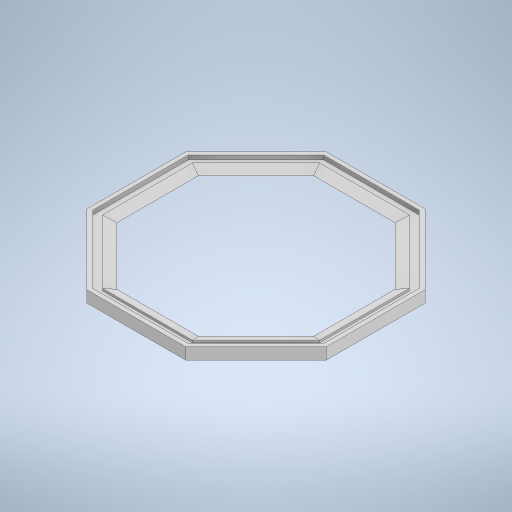
# Autodesk Inventor part: OV-PAM_ring_2
Saved by Autodesk Inventor 2024 (Build 280153000, 153)
## iProperties
Created: 2023-06-19
Part Number: OV-PAM_ring_2
Material: 일반
Document SubType Name: Modeling
Designer: jsw
Density: 1 g/cm^3
Appearance: 기본값
Author: jsw
Autodesk Inventor part; units mm, degrees
ref_plane "YZ Plane" through (0, 0, 0) normal (1, 0, 0) x (0, 1, 0)
ref_plane "XZ Plane" through (0, 0, 0) normal (0, 1, 0) x (-1, 0, 0)
sketch "스케치1" plane through (0, 0, 0) normal (0, 1, 0) x (-1, 0, 0)
  line L0 (-32.5919, 13.5) -> (-13.5, 32.5919)
  line L1 (-13.5, 32.5919) -> (13.5, 32.5919)
  line L2 (13.5, 32.5919) -> (32.5919, 13.5)
  line L3 (32.5919, 13.5) -> (32.5919, -13.5)
  line L4 (32.5919, -13.5) -> (13.5, -32.5919)
  line L5 (13.5, -32.5919) -> (-13.5, -32.5919)
  line L6 (-13.5, -32.5919) -> (-32.5919, -13.5)
  line L7 (-32.5919, -13.5) -> (-32.5919, 13.5)
  line L8 (34.9919, 14.4941) -> (34.9919, -14.4941)
  line L9 (34.9919, -14.4941) -> (14.4941, -34.9919)
  line L10 (14.4941, -34.9919) -> (-14.4941, -34.9919)
  line L11 (-14.4941, -34.9919) -> (-34.9919, -14.4941)
  line L12 (-34.9919, -14.4941) -> (-34.9919, 14.4941)
  line L13 (-34.9919, 14.4941) -> (-14.4941, 34.9919)
  line L14 (-14.4941, 34.9919) -> (14.4941, 34.9919)
  line L15 (14.4941, 34.9919) -> (34.9919, 14.4941)
  point P0 (0, 0)
  point P1 (0, 0)
  point P2 (0, 0)
  dimension "d0" = 27
  dimension "d1" = 2.4
  constraints: 32 end point, 2 coincident, 2 horizontal, 34 other
  measures "d0" distance of L2.end L3.end
  measures "d1" distance between parallel lines of L8 L3
extrude "돌출1" add sketch "스케치1" along normal blind 3.4 contours L0 L1 L2 L3 L4 L5 L6 L7 | L8 L9 L10 L11 L12 L13 L14 L15
sketch "스케치3" plane through (0, 0, 0) normal (0, -1, 0) x (1, 0, 0)
  line L0 (-13.5, 32.5919) -> (13.5, 32.5919)
  line L1 (13.5, 32.5919) -> (32.5919, 13.5)
  line L2 (32.5919, 13.5) -> (32.5919, -13.5)
  line L3 (32.5919, -13.5) -> (13.5, -32.5919)
  line L4 (13.5, -32.5919) -> (-13.5, -32.5919)
  line L5 (-13.5, -32.5919) -> (-32.5919, -13.5)
  line L6 (-32.5919, -13.5) -> (-32.5919, 13.5)
  line L7 (-32.5919, 13.5) -> (-13.5, 32.5919)
  line L8 (-13.9971, 33.7919) -> (13.9971, 33.7919)
  line L9 (13.9971, 33.7919) -> (33.7919, 13.9971)
  line L10 (33.7919, 13.9971) -> (33.7919, -13.9971)
  line L11 (33.7919, -13.9971) -> (13.9971, -33.7919)
  line L12 (13.9971, -33.7919) -> (-13.9971, -33.7919)
  line L13 (-13.9971, -33.7919) -> (-33.7919, -13.9971)
  line L14 (-33.7919, -13.9971) -> (-33.7919, 13.9971)
  line L15 (-33.7919, 13.9971) -> (-13.9971, 33.7919)
  line L16 (-13.1686, 31.7919) -> (13.1686, 31.7919)
  line L17 (13.1686, 31.7919) -> (31.7919, 13.1686)
  line L18 (31.7919, 13.1686) -> (31.7919, -13.1686)
  line L19 (31.7919, -13.1686) -> (13.1686, -31.7919)
  line L20 (13.1686, -31.7919) -> (-13.1686, -31.7919)
  line L21 (-13.1686, -31.7919) -> (-31.7919, -13.1686)
  line L22 (-31.7919, -13.1686) -> (-31.7919, 13.1686)
  line L23 (-31.7919, 13.1686) -> (-13.1686, 31.7919)
  point P0 (0, 0)
  point P1 (0, 0)
  point P2 (0, 0)
  point P3 (0, 0)
  dimension "d8" = 27
  dimension "d9" = 1.2
  dimension "d19" = 0.8
  constraints: 48 end point, 3 coincident, 3 horizontal, 51 other
  measures "d8" distance of L0.start L0.end
  measures "d9" distance between parallel lines of L8 L0
  measures "d19" distance between parallel lines of L16 L0
extrude "돌출3" cut sketch "스케치3" against normal blind 1.2 contours L0 L1 L2 L3 L4 L5 L6 L7 | L8 L9 L10 L11 L12 L13 L14 L15
sketch "스케치4" plane through (0, 3.4, 0) normal (0, 1, 0) x (1, 0, 0)
  line L0 (11.926, -28.7919) -> (-11.926, -28.7919)
  line L1 (-11.926, -28.7919) -> (-28.7919, -11.926)
  line L2 (-28.7919, -11.926) -> (-28.7919, 11.926)
  line L3 (-28.7919, 11.926) -> (-11.926, 28.7919)
  line L4 (-11.926, 28.7919) -> (11.926, 28.7919)
  line L5 (11.926, 28.7919) -> (28.7919, 11.926)
  line L6 (28.7919, 11.926) -> (28.7919, -11.926)
  line L7 (28.7919, -11.926) -> (11.926, -28.7919)
  line L8 (-31.7919, -13.1686) -> (-31.7919, 13.1686) projected
  point P0 (0, 0)
  point P1 (0, 0)
  dimension "d21" = 3
  constraints: 16 end point, 1 coincident, 1 horizontal, 17 other
  measures "d21" distance between parallel lines of L8 L2
extrude "돌출4" cut sketch "스케치4" against normal blind 5
ref_plane "작업 평면1" through (0, 1.7, 0) normal (0, 1, 0) x (1, 0, 0)
sketch "스케치6" plane through (0, 0, 0) normal (0, -1, 0) x (1, 0, 0)
  line L0 (28.7919, -11.926) -> (11.926, -28.7919) projected
  line L1 (11.926, -28.7919) -> (-11.926, -28.7919) projected
  line L2 (-11.926, -28.7919) -> (-28.7919, -11.926) projected
  line L3 (-28.7919, -11.926) -> (-28.7919, 11.926) projected
  line L4 (-28.7919, 11.926) -> (-11.926, 28.7919) projected
  line L5 (-11.926, 28.7919) -> (11.926, 28.7919) projected
  line L6 (11.926, 28.7919) -> (28.7919, 11.926) projected
  line L7 (28.7919, 11.926) -> (28.7919, -11.926) projected
  line L8 (31.7919, 13.1686) -> (13.1686, 31.7919) projected
  line L9 (13.1686, 31.7919) -> (-13.1686, 31.7919) projected
  line L10 (-13.1686, 31.7919) -> (-31.7919, 13.1686) projected
  line L11 (-31.7919, 13.1686) -> (-31.7919, -13.1686) projected
  line L12 (-31.7919, -13.1686) -> (-13.1686, -31.7919) projected
  line L13 (-13.1686, -31.7919) -> (13.1686, -31.7919) projected
  line L14 (13.1686, -31.7919) -> (31.7919, -13.1686) projected
  line L15 (31.7919, -13.1686) -> (31.7919, 13.1686) projected
  point P0 (0, 0)
extrude "돌출7" cut sketch "스케치6" against normal blind 0.6
mirror "미러2" about plane through (0, 1.7, 0) normal (0, 1, 0) of "돌출7", "돌출3"
chamfer "모따기6" distance 1.1 distance2 3 1 edges at (-20.3589, 2.8, -20.3589) measured on face at (-17.548, 2.0667, -23.1699)
chamfer "모따기7" distance 1.1 distance2 3 1 edges at (0, 2.8, -28.7919) measured on face at (3.9753, 1.7, -28.7919)
chamfer "모따기8" distance 1.1 distance2 3 1 edges at (20.3589, 2.8, -20.3589) measured on face at (23.1699, 1.7, -17.548)
chamfer "모따기9" distance 1.1 distance2 3 1 edges at (28.7919, 2.8, 0) measured on face at (28.7919, 1.7, 3.9753)
chamfer "모따기10" distance 1.1 distance2 3 1 edges at (-28.7919, 2.8, 0) measured on face at (-28.7919, 1.7, 3.9753)
chamfer "모따기11" distance 1.1 distance2 3 1 edges at (-20.3589, 2.8, 20.3589) measured on face at (-17.548, 1.7, 23.1699)
chamfer "모따기12" distance 1.1 distance2 3 1 edges at (0, 2.8, 28.7919) measured on face at (3.9753, 1.7, 28.7919)
chamfer "모따기13" distance 1.1 distance2 3 1 edges at (20.3589, 2.8, 20.3589) measured on face at (23.1699, 0.9667, 17.548)
chamfer "모따기14" distance 1.1 distance2 3 1 edges at (-20.3589, 0.6, -20.3589) measured on face at (-17.548, 1.3334, -23.1699)
chamfer "모따기15" distance 1.1 distance2 3 1 edges at (-28.7919, 0.6, 0) measured on face at (-28.7919, 1.3333, 3.9753)
chamfer "모따기16" distance 1.1 distance2 3 1 edges at (-20.3589, 0.6, 20.3589) measured on face at (-17.548, 1.3333, 23.1699)
chamfer "모따기17" distance 1.1 distance2 3 1 edges at (0, 0.6, 28.7919) measured on face at (3.9753, 1.3333, 28.7919)
chamfer "모따기18" distance 1.1 distance2 3 1 edges at (20.3589, 0.6, 20.3589) measured on face at (23.1699, 1.3333, 17.548)
chamfer "모따기19" distance 1.1 distance2 3 1 edges at (28.7919, 0.6, 0) measured on face at (28.7919, 1.3333, -3.9753)
chamfer "모따기20" distance 1.1 distance2 3 1 edges at (20.3589, 0.6, -20.3589) measured on face at (17.548, 1.3333, -23.1699)
chamfer "모따기21" distance 1.1 distance2 3 1 edges at (0, 0.6, -28.7919) measured on face at (-3.9753, 0.9666, -28.7919)
